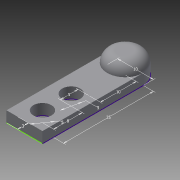
# Autodesk Inventor part: clip_tip(2)
Saved by Autodesk Inventor 2015 (Build 190159000, 159)
## iProperties
Created: 2017-10-03
Part Number: clip_tip(2)
Material: Generic
Document SubType Name: Modeling
Designer: Anshul
Density: 1 g/cm^3
Appearance: Default
Author: Anshul
Autodesk Inventor part; units mm, degrees
ref_plane "YZ Plane" through (0, 0, 0) normal (1, 0, 0) x (0, 1, 0)
ref_plane "XZ Plane" through (0, 0, 0) normal (0, 1, 0) x (-1, 0, 0)
ref_plane "XY Plane" through (0, 0, 0) normal (0, 0, 1) x (1, 0, 0)
sketch "Sketch1" plane through (0, 0, 0) normal (0, 1, 0) x (-1, 0, 0)
  line L0 (0, 0) -> (0, -25)
  line L1 (0, -25) -> (10, -25)
  line L2 (10, -25) -> (10, 0)
  circle A0 centre (5, -25) radius 5
  line L3 (5, -25) -> (5, -15)
  line L4 (5, -15) -> (5, -10)
  circle A1 centre (5, -10) radius 2.5
  line L5 (10, 0) -> (10, 3)
  line L6 (10, 3) -> (0, 3)
  line L7 (0, 3) -> (0, 0)
  line L8 (5, -10) -> (5, -2)
  circle A2 centre (5, -2) radius 2.5
  point P0 (5, 0)
  dimension "d0" = 25
  dimension "d1" = 10
  dimension "d12" = 10
  dimension "d13" = 5
  dimension "d14" = 5
  dimension "d15" = 3
  dimension "d16" = 8
  dimension "d17" = 5
  constraints: 18 end point, 4 perpendicular, 4 vertical, 2 centre point, 2 coincident, 1 horizontal alignment, 1 midpoint, 1 point on line, 2 other
  measures "d0" distance of L0.start L0.end
  measures "d1" distance of L0.end L1.end
  measures "d12" distance of L3.start L3.end
  measures "d13" distance of L3.end L4.end
  measures "d14" diameter of A1
  measures "d15" distance of L2.end L5.end
  measures "d16" distance of L8.start L8.end
  measures "d17" diameter of A2
extrude "Extrusion3" add sketch "Sketch1" along normal blind 3
extrude "Extrusion4" add sketch "Sketch1" along normal blind 6 contours A0 L3 L1 | L1 A0 | L3 A0 L1
fillet "Fillet3" radius 3 1 edges at (0, 6, -25)
body "Solid2"
